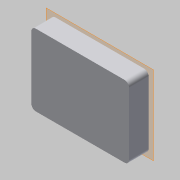
# Autodesk Inventor part: LS2_LEDs_patch
Saved by Autodesk Inventor 2019.3 (Build 233278000, 278)
## iProperties
Created: 2019-04-11
Part Number: LS2_LEDs_patch
Material: Generic
Document SubType Name: Modeling
Designer: Varga Daniel
Density: 1 g/cm^3
Appearance: White - P 1-1 C
Author: Varga Daniel
Autodesk Inventor part; units mm, degrees
ref_plane "YZ Plane" through (0, 0, 0) normal (1, 0, 0) x (0, 1, 0)
ref_plane "XZ Plane" through (0, 0, 0) normal (0, 1, 0) x (-1, 0, 0)
ref_plane "XY Plane" through (0, 0, 0) normal (0, 0, 1) x (1, 0, 0)
ref_plane "Work Plane1" through (0, 0, 0) normal (0, 0, 1) x (1, 0, 0)
sketch "Sketch1" plane through (0, 0, 0) normal (0, 0, 1) x (1, 0, 0)
  line L0 (-13.1, -2.25) -> (-13.1, -7.35) projected
  arc A0 (-13.6, 0.7) -> (-14.3, 0) centre (-13.6, 0) ccw projected
  line L1 (-13.6, 0.7) -> (0, 0.7) projected
  arc A1 (0.7, 0) -> (0, 0.7) centre (0, 0) ccw projected
  line L2 (0.7, 0) -> (0.7, -9.6) projected
  arc A2 (0, -10.3) -> (0.7, -9.6) centre (0, -9.6) ccw projected
  line L3 (0, -10.3) -> (-13.6, -10.3) projected
  arc A3 (-14.3, -9.6) -> (-13.6, -10.3) centre (-13.6, -9.6) ccw projected
  line L4 (-14.3, -9.6) -> (-14.3, 0) projected
  line L5 (-2.25, -9.1) -> (-11.35, -9.1) projected
  arc A4 (-2.25, -9.1) -> (-0.5, -7.35) centre (-2.25, -7.35) ccw projected
  line L6 (-0.5, -2.25) -> (-0.5, -7.35) projected
  arc A5 (-0.5, -2.25) -> (-2.25, -0.5) centre (-2.25, -2.25) ccw projected
  line L7 (-11.35, -0.5) -> (-2.25, -0.5) projected
  arc A6 (-11.35, -0.5) -> (-13.1, -2.25) centre (-11.35, -2.25) ccw projected
  line L8 (-13.1, -7.35) -> (-13.1, -2.25) projected
  arc A7 (-13.1, -7.35) -> (-11.35, -9.1) centre (-11.35, -7.35) ccw projected
  point P0 (0, 0)
extrude "Extrusion1" add sketch "Sketch1" along normal blind 3.01 contours A6 L7 A5 L6 A4 L5 A7 L0 | L1 A1 L2 A2 L3 A3 L4 A0
body "Solid1"
